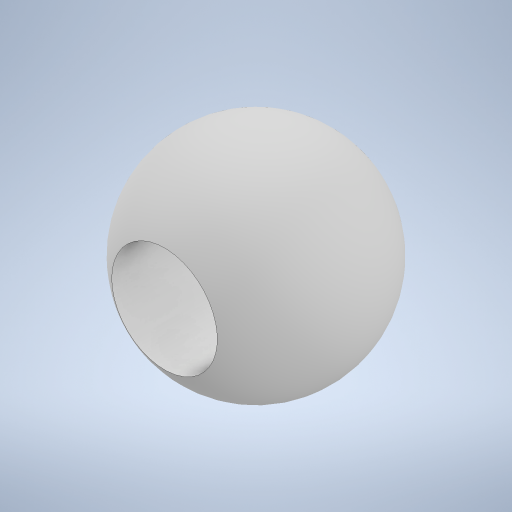
# Autodesk Inventor part: ball
Saved by Autodesk Inventor 2024 (Build 280153000, 153)
## iProperties
Created: 2023-07-07
Part Number: ball
Material: Generic
Document SubType Name: Modeling
Designer: birud
Density: 1 g/cm^3
Appearance: Default
Author: birud
Autodesk Inventor part; units mm, degrees
ref_plane "YZ Plane" through (0, 0, 0) normal (1, 0, 0) x (0, 1, 0)
ref_plane "XZ Plane" through (0, 0, 0) normal (0, 1, 0) x (-1, 0, 0)
ref_plane "XY Plane" through (0, 0, 0) normal (0, 0, 1) x (1, 0, 0)
sketch "Sketch1" plane through (0, 0, 0) normal (0, 0, 1) x (1, 0, 0)
  line L0 (0, 4.445) -> (0, -4.445) projected
  arc A0 (0, 3.175) -> (0, -3.175) centre (0, 0) ccw
  circle A1 centre (0, 0) radius 1.5875
  line L1 (0, 3.175) -> (0, -3.175)
  dimension "d0" = 3.175
  dimension "d1" = 3.175
  constraints: 3 point on circle, 2 centre point, 2 coincident, 2 end point, 2 point on line, 1 collinear
  measures "d0" diameter of A1
  measures "d1" radius of A0
revolve "Revolution1" add sketch "Sketch1" angle 360 about axis through (0, 0, 0) along (0, -1, 0) picked at (-0.4775, -0.3807) contours L0 A1 A0 | L0 A1
extrude "Extrusion1" cut sketch "Sketch1" along normal mid plane 6.35 contours A1 L0 | L0 A1
scale "Scale1" factors (10, 10, 10) then translate (0, 0, 0) bodies 1
body "Solid1"
